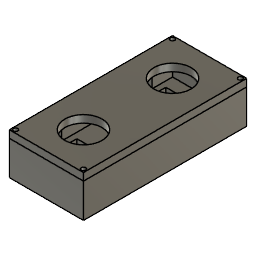
rov_v1 (Autodesk Fusion 360 archive; units mm, degrees)
design "Controller"
part number: 2026-06-03-19-35-21-348
Autodesk Fusion 360 part; units mm, degrees
note: some values were not read from the file. Set by a fixed rule: the direction of a hole.
sketch "Bottom Base" plane through (0, 0, 0) normal (0, 0, 1) x (1, 0, 0)
  line L0 (-74.3735, 55) -> (-124.3735, 55)
  line L1 (-124.3735, 55) -> (-124.3735, -55)
  line L2 (-124.3735, -55) -> (-74.3735, -55)
  line L3 (-74.3735, -55) -> (-74.3735, 55)
  line L4 (-82.3735, 42.5) -> (-116.3735, 42.5)
  line L5 (-116.3735, 42.5) -> (-116.3735, 16.5)
  line L6 (-116.3735, 16.5) -> (-82.3735, 16.5)
  line L7 (-82.3735, 16.5) -> (-82.3735, 42.5)
  line L8 (-82.3735, 42.5) -> (-116.3735, 16.5) construction
  line L9 (-116.3735, 42.5) -> (-82.3735, 16.5) construction
  line L10 (-116.3754, -17.5022) -> (-82.3715, -17.5022)
  line L11 (-82.3715, -17.5022) -> (-82.3715, -43.4978)
  line L12 (-82.3715, -43.4978) -> (-116.3754, -43.4978)
  line L13 (-116.3754, -43.4978) -> (-116.3754, -17.5022)
  line L14 (-116.3754, -17.5022) -> (-82.3715, -43.4978) construction
  line L15 (-82.3715, -17.5022) -> (-116.3754, -43.4978) construction
  line L16 (-82.3735, 42.5) -> (-82.3735, 39.5)
  line L17 (-82.3735, 39.5) -> (-85.3735, 39.5)
  line L18 (-82.3735, 39.5) -> (-111.3735, 39.5)
  line L19 (-124.3735, 37) -> (-124.3735, 24)
  line L20 (-124.3735, -24) -> (-124.3735, -37)
  line L21 (-124.3735, 37) -> (-120, 37)
  line L22 (-120, 37) -> (-120, 24)
  line L23 (-120, 24) -> (-124.3735, 24)
  line L24 (-124.3735, -24) -> (-120, -24)
  line L25 (-120, -24) -> (-120, -37)
  line L26 (-120, -37) -> (-124.3735, -37)
  line L27 (-85.3735, 39.5) -> (-85.3735, 19.25)
  line L28 (-85.3735, 19.25) -> (-111.3735, 19.25)
  line L29 (-99.3735, -30.5) -> (-99.3735, -30)
  line L30 (-99.3735, -30, 0) -> (-99.3735, -30, 15)
  line L31 (-99.3735, 30, 0) -> (-99.3735, 30, 15)
  point P0 (-99.3735, 29.5)
  point P1 (-99.3735, -30.5)
  point P2 (-124.3735, 30.5)
  point P3 (-124.3735, -30.5)
  point P4 (-111.3735, -40.25)
  point P5 (-85.3735, -40.25)
  point P6 (-111.3735, -20)
  point P7 (-85.3735, -20)
  dimension "d1" = 110
  dimension "d2" = 50
  dimension "d10" = 34
  dimension "d11" = 26
  dimension "d14" = 3
  dimension "d15" = 3
  dimension "d16" = 29
  dimension "d26" = 13
  dimension "d62" = 20.25
  dimension "d63" = 26
  dimension "d68" = 15
  constraint horizontal L0
  constraint perpendicular L0 L1
  constraint parallel L0 L2
  constraint parallel L1 L3
  constraint horizontal L4
  constraint perpendicular L4 L5
  constraint parallel L4 L6
  constraint parallel L5 L7
  constraint coincident L8 P0
  constraint coincident L9 P0
  constraint horizontal L10
  constraint perpendicular L10 L11
  constraint parallel L10 L12
  constraint parallel L11 L13
  constraint perpendicular L4 L16
  constraint perpendicular L16 L17
  constraint perpendicular L7 L18
  constraint midpoint L19 P2
  constraint coincident L1 P2
  constraint parallel L1 L19
  constraint midpoint L20 P3
  constraint coincident L1 P3
  constraint parallel L1 L20
  constraint horizontal L21
  constraint vertical L22
  constraint horizontal L23
  constraint horizontal L24
  constraint vertical L25
  constraint horizontal L26
  constraint perpendicular L18 L27
  constraint perpendicular L27 L28
  constraint vertical P0 P1
  measures "d1" distance of L0.end L1.end
  measures "d2" distance of L1.end L2.end
  measures "d10" distance of L5.end L6.end
  measures "d11" distance of L4.end L5.end
  measures "d14" distance of L4.start L16.end
  measures "d15" distance of L16.end L17.end
  measures "d16" distance of L16.end L18.end
  measures "d26" distance of L19.start L19.end
  measures "d62" distance of L17.end L27.end
  measures "d63" distance of L27.end L28.end
extrude "Extrude1" add sketch "Bottom Base" along normal blind 15 and the other way blind 8 contours L0 L1 L2 L3 L21 L22 L23 L24 L25 L26 | L1 L19 L21 L22 L23 | L1 L20 L24 L25 L26 | L4 L5 L6 L7 L16 | L10 L11 L12 L13 makes body 1
sketch "Top Base" plane through (0, 0, 15) normal (0, 0, 1) x (-1, 0, 0)
  line L0 (74.3735, 55) -> (74.3735, -55)
  line L1 (74.3735, -55) -> (124.3735, -55)
  line L2 (124.3735, -55) -> (124.3735, 55)
  line L3 (124.3735, 55) -> (74.3735, 55)
  line L4 (74.3735, 55) -> (78.6161, 50.7574)
  line L5 (74.3735, 55) -> (80.3735, 55) construction
  line L6 (74.3735, -55) -> (78.6161, -50.7574)
  line L7 (74.3735, -55) -> (80.3735, -55) construction
  line L8 (124.3735, -55) -> (120.1308, -50.7574)
  line L9 (124.3735, -55) -> (115.8882, -55) construction
  line L10 (120.1308, -50.7574) -> (78.6161, -50.7574)
  line L11 (78.6161, -50.7574) -> (78.6161, 50.7574)
  line L12 (78.6161, 50.7574) -> (120.1308, 50.7574)
  line L13 (120.1308, 50.7574) -> (120.1308, -50.7574)
  dimension "d32" = 45
  dimension "d33" = 6
  dimension "d34" = 45
  dimension "d35" = 6
  dimension "d37" = 6
  constraint horizontal L5
  constraint coincident L0.start L3.end
  constraint horizontal L7
  constraint coincident L0.end L1.start
  constraint horizontal L9
  constraint coincident L1.end L2.start
  constraint horizontal L10
  constraint vertical L11
  constraint horizontal L12
  constraint vertical L13
  measures "d32" angle of L4 L5
  measures "d33" distance of L0.start L4.end
  measures "d34" angle of L6 L7
  measures "d35" distance of L0.end L6.end
  measures "d37" distance of L1.end L8.end
extrude "Extrude3" cut sketch "Bottom Base" against normal blind 3 contours L4 L5 L6 L7 L16 | L10 L11 L12 L13 bodies 1
extrude "Extrude5" cut sketch "Bottom Base" along normal blind 15 contours L1 L19 L21 L22 L23 bodies 1
extrude "Extrude6" cut sketch "Bottom Base" along normal blind 15 contours L1 L20 L24 L25 L26 bodies 1
extrude "Extrude7" cut sketch "Top Base" against normal blind 15 contours L10 L11 L12 L13 bodies 1
extrude "Extrude8" add sketch "Top Base" along normal blind 5 separate body makes body 2
sketch "Panel Fasteners" plane through (0, 0, 20) normal (0, 0, 1) x (-1, 0, 0)
  line L0 (124.3735, 55) -> (74.3735, 55)
  line L1 (74.3735, 55) -> (74.3735, -55)
  line L2 (74.3735, -55) -> (124.3735, -55)
  line L3 (124.3735, -55) -> (124.3735, 55)
  line L4 (74.3735, 55) -> (76.4948, 52.8787)
  line L5 (74.3735, 55) -> (77.3735, 55) construction
  line L6 (74.3735, -55) -> (76.4948, -52.8787)
  line L7 (74.3735, -55) -> (77.3735, -55) construction
  line L8 (124.3735, -55) -> (122.2521, -52.8787)
  line L9 (124.3735, -55) -> (121.3735, -55) construction
  line L10 (124.3735, 55) -> (122.2521, 52.8787)
  line L11 (124.3735, 55) -> (121.3735, 55) construction
  dimension "d47" = 45
  dimension "d48" = 3
  dimension "d49" = 45
  dimension "d50" = 3
  dimension "d54" = 45
  dimension "d55" = 3
  dimension "d56" = 45
  dimension "d57" = 3
  constraint horizontal L5
  constraint coincident L0.end L1.start
  constraint horizontal L7
  constraint coincident L1.end L2.start
  constraint horizontal L9
  constraint coincident L2.end L3.start
  constraint horizontal L11
  constraint coincident L0.start L3.end
  measures "d47" angle of L4 L5
  measures "d48" distance of L0.end L4.end
  measures "d49" angle of L6 L7
  measures "d50" distance of L1.end L6.end
  measures "d54" angle of L8 L9
  measures "d55" distance of L2.end L8.end
  measures "d56" angle of L10 L11
  measures "d57" distance of L0.start L10.end
hole "Hole4" at (-76.4948, -52.8787, 20) at (-122.2521, -52.8787, 20) at (-122.2521, 52.8787, 20) at (-76.4948, 52.8787, 20) direction (0, 0, -1) diameter 3 depth 12 tip angle 180 bodies 1 2
hole "Hole5" at (-111.3735, 19.25, 0) at (-111.3735, 39.5, 0) at (-85.3735, 39.5, 0) at (-85.3735, 19.25, 0) at (-111.3735, -20, 0) at (-111.3735, -40.25, 0) at (-85.3735, -40.25, 0) at (-85.3735, -20, 0) direction (0, 0, -1) diameter 3 depth 6 tip angle 180 bodies 1
hole "Hole6" at (-99.3735, -30, 15) at (-99.3735, 30, 15) direction (0, 0, 1) diameter 25 depth 5 tip angle 180 bodies 2
named bodies: "Controller Base", "Joystick Panel"

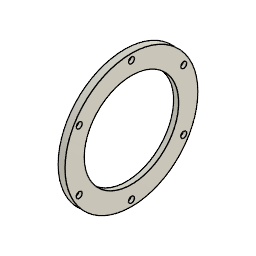
design "Front Brace"
part number: 2026-03-16-16-23-55-166
Autodesk Fusion 360 part; units mm, degrees
sketch "Base" plane through (0, 0, 0) normal (1, 0, 0) x (0, 1, 0)
  circle A0 centre (0, 0) radius 47.625
  circle A1 centre (0, 0) radius 40.64
  circle A2 centre (0, 0) radius 60.325
  dimension "d86" = 95.25
  dimension "d87" = 81.28
  dimension "d99" = 120.65
  constraint coincident A0.centre A1.centre
  constraint concentric A0 A1
  constraint concentric A1 A2
  measures "d86" diameter of A0
  measures "d87" diameter of A1
  measures "d99" diameter of A2
extrude "Extrude1" add sketch "Base" along normal blind 1.778 contours A0 makes body 1
move_body "Move1" bodies 1 to x (1, 0, 0) y (0, 1, 0) z (0, 0, 1) at (254, 228.6, -50.8)
move_body "Move2" bodies 1 to x (1, 0, 0) y (0, 1, 0) z (0, 0, 1) at (45.72, -53.34, 50.8)
move_body "Move3" bodies 1 to x (1, 0, 0) y (0, 1, 0) z (0, 0, 1) at (-1.2446, 0, 0)
extrude "Extrude2" add sketch "Base" along normal blind 3.556 separate body contours A2 makes body 2
move_body "Move4" bodies 2 to x (1, 0, 0) y (0, 1, 0) z (0, 0, 1) at (297.18, 175.26, 0)
move_body "Move5" bodies 2 to x (1, 0, 0) y (0, 1, 0) z (0, 0, 1) at (-0.4826, 0, 0)
combine "Combine1" operation add target body 1 tool bodies 2
move_body "Move6" bodies 1 to x (1, 0, 0) y (0, 1, 0) z (0, 0, 1) at (63.5, 0, 0)
extrude "Extrude3" cut 1 faces at (360.1974, 230.9498, -5.363) along direction (1, 0, 0) blind 0.1778 on bodies 1 bodies 1
move_body "Move7" bodies 1 to x (1, 0, 0) y (0, 1, 0) z (0, 0, 1) at (-63.5, 0, 0)
move_body "Move8" bodies 1 to x (1, 0, 0) y (0, 1, 0) z (0, 0, 1) at (50.8, 0, 0)
move_body "Move9" bodies 1 to x (1, 0, 0) y (0, 1, 0) z (0, 0, 1) at (-152.4, 0, 0)
move_body "Move10" bodies 1 to x (1, 0, 0) y (0, 1, 0) z (0, 0, 1) at (0, 0.1778, 0)
move_body "Move11" bodies 1 to x (1, 0, 0) y (0, 1, 0) z (0, 0, 1) at (0, -0.0508, 0)
move_body "Move12" bodies 1 to x (1, 0, 0) y (0, 1, 0) z (0, 0, 1) at (127, 0, 0)
move_body "Move13" bodies 1 to x (1, 0, 0) y (0, 1, 0) z (0, 0, 1) at (-50.8, 0, 0)
hole "Hole1" at (274.8534, 121.2694, -0.0106) direction (-1, 0, 0) diameter 3.81 depth 20.6375 tip angle 180 bodies 1
pattern_circular "C-Pattern2" count 5 over 360 about axis through (274.8534, 175.387, 0) along (1, 0, 0) of "Hole1"
move_body "Move18" bodies 1 to x (1, 0, 0) y (0, 1, 0) z (0, 0, 1) at (63.5, 0, 0)
move_body "Move19" bodies 1 to x (1, 0, 0) y (0, 1, 0) z (0, 0, 1) at (-63.5, 0, 0)
move_body "Move20" bodies 1 to x (1, 0, 0) y (0, 1, 0) z (0, 0, 1) at (63.5, 0, 0)
move_body "Move21" bodies 1 to x (1, 0, 0) y (0, 1, 0) z (0, 0, 1) at (-63.5, 0, 0)
move_body "Move22" bodies 1 to x (1, 0, 0) y (0, 1, 0) z (0, 0, 1) at (63.5, 0, 0)
move_body "Move23" bodies 1 to x (1, 0, 0) y (0, 1, 0) z (0, 0, 1) at (-63.5, 0, 0)
move_body "Move24" bodies 1 to x (1, 0, 0) y (0, 1, 0) z (0, 0, 1) at (-68.58, 0, 0)
move_body "Align1" bodies 1 to x (1, 0, 0) y (0, 1, 0) z (0, 0, 1) at (-202.8952, 0, 0)
move_body "Align2" bodies 1 to x (1, 0, 0) y (0, 1, 0) z (0, 0, 1) at (-1.6002, -175.387, 0)
move_body "Align3" bodies 1 to x (1, 0, 0) y (0, 1, 0) z (0, 0, 1) at (1.6002, 0, 0)
delete_face "DeleteFace1" 1 faces at (2.2521, -18.5135, 50.7874) on bodies 1
delete_face "DeleteFace2" 1 faces at (2.2521, 42.5807, 33.3015) on bodies 1
delete_face "DeleteFace3" 1 faces at (2.2521, 44.8298, -30.2059) on bodies 1
delete_face "DeleteFace4" 1 faces at (2.2521, -54.0227, -1.9132) on bodies 1
delete_face "DeleteFace5" 1 faces at (2.2521, -14.8744, -51.9698) on bodies 1
sketch "Outer Ring" plane through (3.3782, 0, 0) normal (1, 0, 0) x (0, 1, 0)
  circle A0 centre (0, 0) radius 60.325
  circle A1 centre (0, 0) radius 40.64
  circle A2 centre (0, 0) radius 60.325
  circle A3 centre (0, 0) radius 57.263
  dimension "d1" = 120.65
  dimension "d2" = 114.526
  constraint concentric A0 A2
  constraint concentric A2 A3
  measures "d1" diameter of A2
  measures "d2" diameter of A3
extrude "Extrude4" cut sketch "Outer Ring" against normal blind 10 contours A0 A2 bodies 1
sketch "Extension" plane through (3.3782, 0, 0) normal (1, 0, 0) x (0, 1, 0)
  circle A0 centre (0, 0) radius 57.263
  circle A1 centre (0, 0) radius 40.64
  circle A2 centre (0, 0) radius 40.64
  circle A3 centre (0, 0) radius 57.263
  dimension "d6" = 81.28
  dimension "d7" = 114.526
  constraint concentric A0 A2
  constraint concentric A0 A3
  measures "d6" diameter of A2
  measures "d7" diameter of A3
extrude "Extrude5" add sketch "Extension" along normal blind 2.622 bodies 1
sketch "Fastener Hole" plane through (6.0002, 0, 0) normal (1, 0, 0) x (0, 1, 0)
  circle A0 centre (0, 0) radius 40.64
  circle A1 centre (0, 0) radius 57.263
  line L0 (0, 0) -> (0, 52)
  dimension "d10" = 52
  constraint coincident A0.centre A1.centre
  constraint vertical L0
  measures "d10" distance of A0.centre L0.end
hole "Hole2" at (6.0002, 0, 52) direction (-1, 0, 0) diameter 3 depth 7 tip angle 180 counterbore diameter 5.1 counterbore depth 3 bodies 1
pattern_circular "C-Pattern3" count 6 over 360 about axis through (1.75, 0, 0) along (1, 0, 0) of "Hole2"
pattern_circular "C-Pattern1" [suppressed]
move_body "Move14" [suppressed]
move_body "Move15" [suppressed]
move_body "Move16" [suppressed]
move_body "Move17" [suppressed]
named bodies: "Front Brace"
